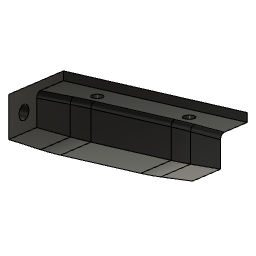
Back mount attachment (Autodesk Fusion 360 archive; units mm, degrees)
design "Back mount attachment" references "Micro Delta Rework", "Plaque de support"
Autodesk Fusion 360 part; units mm, degrees
note: some values were not read from the file. Set by a fixed rule: which face or edge a step refers to.
derive "Dérivé à partir de Micro Delta Rework v14" from "Micro Delta Rework v14"
derive "Dérivé à partir de Plaque de support v19" from "Plaque de support v19"
box "BoitePrimitive1" add length 25 width 25 height 110 placed x (0, 1, 0) y (-1, 0, 0) z (0, 0, 1) at (25, 0, 0)
hole "Perçage1" at (12.5, 12.5, 110) direction (0, 0, -1) diameter 8.2 end through all
sketch "Esquisse8" plane through (25, 0, 0) normal (1, 0, 0) x (0, 0, -1)
  line L0 (-110, 0) -> (0, 0)
  line L1 (0, 0) -> (0, 25)
  line L2 (0, 25) -> (-110, 25)
  line L3 (-110, 25) -> (-110, 0)
  line L4 (-110, 20) -> (0, 20)
  dimension "base_l" = 25
  dimension "tige_diam" = 8
  dimension "tige_jeu" = 0.2
  dimension "fixation_ep" = 5
  dimension "fixation_prof" = 20
  dimension "vis_diam" = 6
  dimension "vis_jeu" = 0.6
  dimension "plaque0_l1_Ref" = 160
  dimension "plaque0_l2_Ref" = 95
  dimension "plaque0_l1_Ref_Ref" = 160
  dimension "plaque0_l2_Ref_Ref" = 95
  dimension "support_chanf_Ref" = 25
  dimension "d43" = 5
  dimension "haut_ep_Ref" = 17
  dimension "plaque_ep_Ref" = 2.1
  dimension "haut_conge_Ref" = 3
  constraint coincident L3 L4.start
  constraint coincident L1 L4.end
  constraint perpendicular L1 L4
  measures "d43" distance of L2 L4
extrude "Extrusion2" add sketch "Esquisse8" along normal blind 20 contours L1 L2 L3 L4
sketch "Esquisse9" plane through (0, 20, 0) normal (0, -1, 0) x (1, 0, 0)
  line L0 (25, 110) -> (25, 0)
  line L1 (25, 0) -> (45, 0)
  line L2 (45, 0) -> (45, 110)
  line L3 (45, 110) -> (25, 110)
  line L4 (45, 55) -> (25, 55) construction
  line L5 (25, 110) -> (45, 55) construction
  line L6 (45, 110) -> (25, 55) construction
  line L7 (25, 55) -> (45, 0) construction
  line L8 (45, 55) -> (25, 0) construction
  circle A0 centre (35, 82.5) radius 3.3
  circle A1 centre (35, 27.5) radius 3.3
  dimension "d46" = 6.6
  dimension "d47" = 6.6
  constraint midpoint L2 L4.start
  constraint midpoint L0 L4.end
  constraint coincident L0.start L3.end
  constraint coincident L2.end L3.start
  constraint coincident L1.end L2.start
  constraint coincident L0.end L1.start
  constraint midpoint L5 A0.centre
  constraint midpoint L8 A1.centre
  measures "d46" diameter of A0
  measures "d47" diameter of A1
extrude "Extrusion3" cut sketch "Esquisse9" against normal through all contours A0 | A1
chamfer "Chanfrein5" distance 2 distance2 25 4 edges at (25, 10, 110) (25, 10, 0) (12.5, 0, 110) (12.5, 0, 0) measured on face at (2.8038, 12.6021, 110) measured on face at (2.8038, 12.3979, 0) measured on face at (2.8038, 12.6021, 110) measured on face at (2.8038, 12.3979, 0)
fillet "Congé3" radius 150 4 edges at (25, 10, 85) (12.5, 0, 85) (25, 10, 25) (12.5, 0, 25)
fillet "Congé4" radius 3 5 edges at (23.7611, 20, 9.5143) (24.8805, 20, 25.0048) (25, 20, 55) (24.8805, 20, 84.9952) (23.7611, 20, 100.4857)
equation "base_l = 25 mm"
equation "d4 = plaque0_l1_Ref - support_chanf_Ref * 2"
equation "tige_diam = 8 mm"
equation "tige_jeu = 0.2 mm"
equation "d10 = tige_diam + tige_jeu"
equation "fixation_ep = 5 mm"
equation "fixation_prof = 20 mm"
equation "vis_diam = 6 mm"
equation "vis_jeu = 0.6 mm"
equation "d43 = fixation_ep"
equation "d44 = fixation_prof"
equation "d46 = vis_diam + vis_jeu"
equation "d47 = vis_diam + vis_jeu"
equation "d50 = base_l"
named bodies: "Back mount attachment"

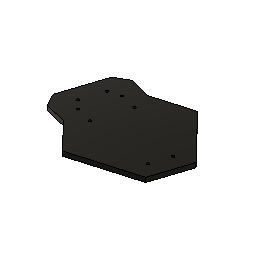
design "Plaque de support" references "Micro Delta Rework"
Autodesk Fusion 360 part; units mm, degrees
derive "Dérivé à partir de Micro Delta Rework v14" from "Micro Delta Rework v14"
sketch "Esquisse1" plane through (0, 0, 0) normal (0, 1, 0) x (1, 0, 0)
  line L0 (0, 0) -> (160, 0)
  line L1 (0, 0) -> (-47.5, 82.2724)
  line L2 (0, 0) -> (95, 0) construction
  line L3 (-47.5, 82.2724) -> (32.5, 220.8365)
  line L4 (-47.5, 82.2724) -> (112.5, 82.2724) construction
  line L5 (160, 0) -> (207.5, 82.2724)
  line L6 (160, 0) -> (255, 0) construction
  line L7 (207.5, 82.2724) -> (127.4604, 220.8136)
  line L8 (207.5, 82.2724) -> (367.5, 82.2724) construction
  line L9 (127.4604, 220.8136) -> (32.5, 220.8365)
  dimension "d3" = 160
  dimension "d4" = 120
  dimension "d5" = 95
  dimension "d6" = 60
  dimension "d7" = 160
  dimension "d8" = 60
  dimension "d9" = 95
  dimension "d10" = 120.016
  dimension "d11" = 160
  constraint coincident L0.start L1.start
  constraint horizontal L0
  constraint horizontal L2
  constraint horizontal L4
  constraint horizontal L6
  constraint horizontal L8
  measures "d3" distance of L0.start L0.end
  measures "d4" angle of L1 L2
  measures "d5" distance of L0.start L1.end
  measures "d6" angle of L3 L4
  measures "d7" distance of L1.end L3.end
  measures "d8" angle of L5 L6
  measures "d9" distance of L0.end L5.end
  measures "d10" angle of L7 L8
  measures "d11" distance of L5.end L7.end
extrude "Extrusion1" add sketch "Esquisse1" along normal blind 10.12
extrude "Extrusion2" add 1 faces at (-20.8333, 3.3733, -128.4604) along direction (-0.866025, 0, -0.5) blind 80
chamfer "Chanfrein1" distance 25 angle 45 2 edges at (-36.782, 5.06, -260.8365) (-116.782, 5.06, -122.2724)
sketch "Esquisse2" plane through (0, 10.12, 0) normal (0, 1, 0) x (-1, 0, 0)
  line L0 (104.282, -143.923) -> (95.1314, -109.7724)
  line L1 (95.1314, -109.7724) -> (47.5, -82.2724)
  line L2 (47.5, -82.2724) -> (0, 0)
  line L3 (0, 0) -> (-160, 0)
  line L4 (-160, 0) -> (-207.5, -82.2724)
  line L5 (-207.5, -82.2724) -> (-127.4604, -220.8136)
  line L6 (-127.4604, -220.8136) -> (-32.5, -220.8365)
  line L7 (-32.5, -220.8365) -> (15.1314, -248.3365)
  line L8 (15.1314, -248.3365) -> (49.282, -239.1858)
  line L9 (49.282, -239.1858) -> (104.282, -143.923)
  line L10 (97.782, -155.1814) -> (-162.75, -4.7631) construction
  line L11 (55.782, -227.9275) -> (-204.75, -77.5093) construction
  line L12 (-15.1795, -230.8365) -> (64.8205, -92.2724) construction
  circle A0 centre (45.8205, -125.1814) radius 3.025
  circle A1 centre (3.8205, -197.9275) radius 3.025
  line L13 (-63.4246, -231.3994) -> (35.087, -60.7724) construction
  circle A2 centre (9.8805, -104.4314) radius 3.025
  circle A3 centre (-32.1195, -177.1775) radius 3.025
  line L14 (6.4495, -243.324) -> (86.4495, -104.7599) construction
  line L15 (90.5195, -167.7604) -> (-170.0125, -17.3422) construction
  line L16 (63.0445, -215.3485) -> (-197.4875, -64.9303) construction
  circle A4 centre (60.187, -150.2479) radius 3.025
  circle A5 centre (32.712, -197.836) radius 3.025
  line L17 (76.782, -191.5544) -> (-183.75, -41.1362) construction
  line L18 (-119.5855, 0) -> (-187.2861, -117.2609) construction
  line L19 (-160, 0) -> (-153.4358, -58.6304) construction
  line L20 (-153.4358, -58.6304) -> (-207.5, -82.2724) construction
  line L21 (-160, 0) -> (-129.6891, -17.5) construction
  line L22 (-207.5, -82.2724) -> (-177.1891, -99.7724) construction
  line L23 (-177.1891, -99.7724) -> (-183.75, -41.1362) construction
  line L24 (-183.75, -41.1362) -> (-129.6891, -17.5) construction
  line L25 (-156.7196, -29.3181) -> (-141.5641, -38.0681) construction
  line L26 (-180.4679, -70.4514) -> (-165.3124, -79.2014) construction
  circle A6 centre (-141.5641, -38.0681) radius 3.025
  circle A7 centre (-165.3124, -79.2014) radius 3.025
  dimension "d24" = 38
  dimension "d26" = 38
  dimension "d28" = 60
  dimension "d30" = 6.05
  dimension "d31" = 6.05
  dimension "d39" = 41.5
  dimension "d40" = 6.05
  dimension "d43" = 6.05
  dimension "d46" = 35.025
  dimension "d49" = 27.525
  dimension "d50" = 27.525
  dimension "d51" = 6.05
  dimension "d52" = 6.05
  dimension "d53" = 35
  dimension "d54" = 6.05
  dimension "d55" = 6.05
  constraint coincident L9 L10.start
  constraint coincident L4 L10.end
  constraint perpendicular L4 L10
  constraint coincident L9 L11.start
  constraint coincident L4 L11.end
  constraint perpendicular L4 L11
  constraint coincident L7 L12.start
  constraint coincident L1 L12.end
  constraint perpendicular L1 L12
  constraint coincident L10 A0.centre
  constraint coincident L12 A0.centre
  constraint coincident L12 A1.centre
  constraint coincident L11 A1.centre
  constraint coincident L2 L13.end
  constraint parallel L12 L13
  constraint coincident L13 A2.centre
  constraint coincident L10 A2.centre
  constraint coincident L11 A3.centre
  constraint coincident L13 A3.centre
  constraint coincident L7 L14.start
  constraint coincident L1 L14.end
  constraint perpendicular L1 L14
  constraint coincident L9 L15.start
  constraint coincident L4 L15.end
  constraint perpendicular L4 L15
  constraint coincident L9 L16.start
  constraint coincident L4 L16.end
  constraint perpendicular L4 L16
  constraint coincident L14 A4.centre
  constraint coincident L15 A4.centre
  constraint coincident L14 A5.centre
  constraint coincident L16 A5.centre
  constraint midpoint L9 L17.start
  constraint midpoint L4 L17.end
  constraint coincident L3 L18.start
  constraint coincident L5 L18.end
  constraint parallel L4 L18
  constraint coincident L3.end L4.start
  constraint midpoint L18 L19.end
  constraint coincident L4.end L5.start
  constraint coincident L18 L21.end
  constraint perpendicular L18 L21
  constraint coincident L18 L22.end
  constraint perpendicular L18 L22
  constraint midpoint L24 L25.start
  constraint coincident L18 L25.end
  constraint perpendicular L18 L25
  constraint midpoint L20 L26.start
  constraint coincident L18 L26.end
  constraint perpendicular L18 L26
  constraint coincident L25.end A6.centre
  constraint coincident L26.end A7.centre
  measures "d24" distance of L1 L10
  measures "d26" distance of L7 L11
  measures "d28" distance of L9 L12
  measures "d30" diameter of A0
  measures "d31" diameter of A1
  measures "d39" distance of L12 L13
  measures "d40" diameter of A2
  measures "d43" diameter of A3
  measures "d46" distance of L9 L14
  measures "d49" distance of L0.start L15
  measures "d50" distance of L8.end L16
  measures "d51" diameter of A4
  measures "d52" diameter of A5
  measures "d53" distance of L4 L18
  measures "d54" diameter of A6
  measures "d55" diameter of A7
extrude "Extrusion3" cut sketch "Esquisse2" against normal through all contours A0 | A1 | A2 | A3 | A4 | A5 | A6 | A7
equation "plaque0_l1_Ref = 160 mm"
equation "plaque0_l2_Ref = 95 mm"
equation "d3 = plaque0_l1_Ref"
equation "d5 = plaque0_l2_Ref"
equation "d7 = plaque0_l1_Ref"
equation "d9 = plaque0_l2_Ref"
equation "d11 = plaque0_l1_Ref"
equation "plaque_ep = 10.12 mm"
equation "d13 = plaque_ep"
equation "d15 = support_prof"
equation "d17 = support_chanf"
equation "support_prof = 80 mm"
equation "support_chanf = 25 mm"
equation "haut_ep_Ref = 17 mm"
equation "plaque_ep_Ref = 2.1 mm"
equation "haut_conge_Ref = 3 mm"
equation "d24 = trou_butée_x"
equation "trou_butée_x = 38 mm"
equation "d26 = trou_butée_x"
equation "trou_butée_y = 60 mm"
equation "d28 = trou_butée_y"
equation "trou_diam = 6.05 mm"
equation "d30 = trou_diam"
equation "d31 = trou_diam"
equation "trou_butée_entraxe = 41.5 mm"
equation "d39 = trou_butée_entraxe"
equation "d40 = trou_diam"
equation "d43 = trou_diam"
equation "trou_glissière_y = 35.025 mm"
equation "trou_glissière_entraxe = 55 mm"
equation "d46 = trou_glissière_y"
equation "trou_glissière_x = 27.525 mm"
equation "d49 = trou_glissière_x"
equation "d50 = trou_glissière_x"
equation "d51 = trou_diam"
equation "d52 = trou_diam"
equation "d54 = trou_diam"
equation "d55 = trou_diam"

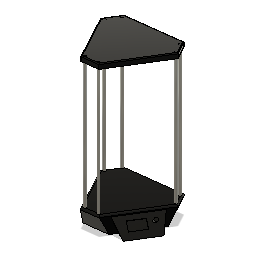
design "Micro Delta Rework"
Autodesk Fusion 360 part; units mm, degrees
sketch "Esquisse1" plane through (0, 0, 0) normal (0, 1, 0) x (1, 0, 0)
  line L0 (0, 0) -> (160, 0)
  line L1 (0, 0) -> (-47.5, 82.2724)
  line L2 (0, 0) -> (95, 0) construction
  line L3 (160, 0) -> (207.5, 82.2724)
  line L4 (160, 0) -> (255, 0) construction
  line L5 (-47.5, 82.2724) -> (32.5, 220.8365)
  line L6 (-47.5, 82.2724) -> (112.5, 82.2724) construction
  line L7 (207.5, 82.2724) -> (127.5, 220.8365)
  line L8 (207.5, 82.2724) -> (367.5, 82.2724) construction
  line L9 (127.5, 220.8365) -> (32.5, 220.8365)
  line L10 (-7.5, 151.5544) -> (183.75, 41.1362) construction
  line L11 (80, 0) -> (80, 220.8365) construction
  line L12 (25, -46) -> (135, -46) construction
  line L13 (5, 0) -> (155, 0)
  circle A0 centre (3.4641, 26) radius 6
  circle A1 centre (156.5359, 26) radius 6
  circle A2 centre (183.2513, 72.2724) radius 6
  circle A3 centre (106.7154, 204.8365) radius 6
  circle A4 centre (53.2846, 204.8365) radius 6
  circle A5 centre (-23.2513, 72.2724) radius 6
  line L14 (18.4752, 0) -> (-38.2624, 98.2724) construction
  line L15 (135.9202, -9.7075) -> (198.2624, 98.2724) construction
  line L16 (23.2624, 204.8365) -> (136.7376, 204.8365) construction
  line L17 (-15.0111, 26) -> (175.0111, 26) construction
  line L18 (192.4889, 56.2724) -> (97.4778, 220.8365) construction
  line L19 (-32.4889, 56.2724) -> (62.5222, 220.8365) construction
  point P0 (80, 101.0363)
  point P1 (80, 0)
  point P2 (80, -46)
  dimension "d1" = 160
  dimension "d2" = 120
  dimension "d3" = 95
  dimension "d4" = 95
  dimension "d5" = 60
  dimension "d6" = 60
  dimension "d7" = 160
  dimension "d8" = 120
  dimension "d9" = 160
  dimension "d62" = 110
  dimension "d63" = 150
  dimension "d64" = 46
  dimension "d98" = 12
  dimension "d99" = 12
  dimension "d100" = 12
  dimension "d101" = 12
  dimension "d102" = 12
  dimension "d103" = 12
  dimension "d104" = 16
  dimension "d105" = 16
  dimension "d106" = 16
  dimension "d107" = 26
  dimension "d108" = 26
  dimension "d109" = 26
  constraint coincident L0.start L1.start
  constraint horizontal L0
  constraint horizontal L2
  constraint horizontal L4
  constraint horizontal L6
  constraint horizontal L8
  constraint midpoint L5 L10.start
  constraint midpoint L3 L10.end
  constraint midpoint L0 P1
  constraint midpoint L9 L11.end
  constraint coincident L11 P0
  constraint coincident L10 P0
  constraint horizontal L12
  constraint horizontal L13
  constraint midpoint L13 P1
  constraint coincident L11 P1
  constraint midpoint L12 P2
  constraint coincident L11 P2
  constraint collinear L0 L13
  constraint coincident L2 L14.start
  constraint coincident L5 L14.end
  constraint coincident L7 L15.end
  constraint coincident L5 L16.start
  constraint coincident L7 L16.end
  constraint parallel L9 L16
  constraint parallel L1 L14
  constraint parallel L3 L15
  constraint coincident L1 L17.start
  constraint coincident L3 L17.end
  constraint coincident L3 L18.start
  constraint coincident L9 L18.end
  constraint coincident L1 L19.start
  constraint coincident L9 L19.end
  constraint parallel L0 L17
  constraint parallel L7 L18
  constraint parallel L5 L19
  constraint coincident A0.centre L17
  constraint coincident A0.centre L14
  constraint coincident A5.centre L14
  constraint coincident A5.centre L19
  constraint coincident A4.centre L19
  constraint coincident A4.centre L16
  constraint coincident A3.centre L18
  constraint coincident A3.centre L16
  constraint coincident A1.centre L15
  constraint coincident A1.centre L17
  constraint coincident A2.centre L18
  constraint coincident A2.centre L15
  measures "d1" distance of L0.start L0.end
  measures "d2" angle of L1 L2
  measures "d3" distance of L0.start L1.end
  measures "d4" distance of L0.end L3.end
  measures "d5" angle of L3 L4
  measures "d6" angle of L5 L6
  measures "d7" distance of L1.end L5.end
  measures "d8" angle of L7 L8
  measures "d9" distance of L3.end L7.end
  measures "d62" distance of L12.start L12.end
  measures "d63" distance of L13.start L13.end
  measures "d64" distance of L12 L13
  measures "d98" diameter of A0
  measures "d99" diameter of A1
  measures "d100" diameter of A2
  measures "d101" diameter of A3
  measures "d102" diameter of A4
  measures "d103" diameter of A5
  measures "d104" distance of L1 L14
  measures "d105" distance of L3 L15
  measures "d106" distance of L9 L16
  measures "d107" distance of L2 L17
  measures "d108" distance of L7 L18
  measures "d109" distance of L5 L19
ref_plane "Plan de construction1" through (0, 60, 0) normal (0, 1, 0) x (0, 0, 1)
sketch "Esquisse2" plane through (0, 60, 0) normal (0, 1, 0) x (1, 0, 0)
  line L0 (-30, 0) -> (190, 0)
  line L1 (-30, 0) -> (-62.5, 56.2917)
  line L2 (-30, 0) -> (35, 0) construction
  line L3 (-62.5, 56.2917) -> (47.5, 246.8172)
  line L4 (-62.5, 56.2917) -> (157.5, 56.2917) construction
  line L5 (190, 0) -> (222.5, 56.2917)
  line L6 (190, 0) -> (255, 0) construction
  line L7 (222.5, 56.2917) -> (112.5, 246.8172)
  line L8 (222.5, 56.2917) -> (442.5, 56.2917) construction
  line L9 (112.5, 246.8172) -> (47.5, 246.8172)
  line L10 (206.25, 28.1458) -> (-7.5, 151.5544) construction
  line L11 (80, 0) -> (80, 246.8172) construction
  line L12 (-56.7265, 66.2917) -> (-18.453, 0) construction
  line L13 (41.7265, 236.8172) -> (118.2735, 236.8172) construction
  line L14 (178.453, 0) -> (216.7265, 66.2917) construction
  circle A0 centre (-25.3812, 12) radius 5
  circle A1 centre (-49.7983, 54.2917) radius 5
  circle A2 centre (184.0544, 9.702) radius 5
  circle A3 centre (206.8348, 49.1587) radius 5
  circle A4 centre (55.5829, 236.8172) radius 5
  circle A5 centre (104.4171, 236.8172) radius 5
  point P0 (80, 101.0363)
  point P1 (80, 101.0363)
  dimension "d18" = 220
  dimension "d19" = 120
  dimension "d20" = 65
  dimension "d21" = 60
  dimension "d22" = 220
  dimension "d23" = 60
  dimension "d24" = 65
  dimension "d25" = 120
  dimension "d26" = 220
  dimension "d43" = 10
  dimension "d44" = 10
  dimension "d45" = 10
  dimension "d47" = 10
  dimension "d48" = 10
  dimension "d49" = 10
  dimension "d50" = 10
  dimension "d51" = 10
  dimension "d52" = 10
  dimension "d53" = 12
  dimension "d54" = 12
  dimension "d55" = 12
  dimension "d56" = 12
  constraint horizontal L0
  constraint horizontal L2
  constraint horizontal L4
  constraint horizontal L6
  constraint horizontal L8
  constraint midpoint L5 L10.start
  constraint midpoint L3 L10.end
  constraint midpoint L0 L11.start
  constraint midpoint L9 L11.end
  constraint coincident L10 P1
  constraint coincident L11 P1
  constraint coincident P1 P0
  constraint coincident L3 L12.start
  constraint coincident L2 L12.end
  constraint coincident L3 L13.start
  constraint coincident L7 L13.end
  constraint coincident L0 L14.start
  constraint coincident L7 L14.end
  constraint parallel L1 L12
  constraint parallel L9 L13
  constraint parallel L5 L14
  constraint coincident L12 A0.centre
  constraint coincident L12 A1.centre
  constraint coincident L14 A2.centre
  constraint coincident L14 A3.centre
  constraint coincident L13 A4.centre
  constraint coincident L13 A5.centre
  measures "d18" distance of L0.start L0.end
  measures "d19" angle of L1 L2
  measures "d20" distance of L0.start L1.end
  measures "d21" angle of L3 L4
  measures "d22" distance of L1.end L3.end
  measures "d23" angle of L5 L6
  measures "d24" distance of L0.end L5.end
  measures "d25" angle of L7 L8
  measures "d26" distance of L5.end L7.end
  measures "d43" distance of L1 L12
  measures "d44" distance of L5 L14
  measures "d45" distance of L9 L13
  measures "d47" diameter of A0
  measures "d48" diameter of A1
  measures "d49" diameter of A2
  measures "d50" diameter of A3
  measures "d51" diameter of A4
  measures "d52" diameter of A5
  measures "d53" distance of L3 A4.centre
  measures "d54" distance of L7 A5.centre
  measures "d55" distance of L2 A0.centre
  measures "d56" distance of L3 A1.centre
loft "Lissage1" add profiles "Esquisse1", "Esquisse2" section 1 contours L0 L1 L3 L5 L7 L9 L13 | A0 | A1 | A2 | A3 | A4 | A5 section 2 contours L0 L1 L3 L5 L7 L9 | A0 | A1 | A2 | A3 | A4 | A5 makes body 1
ref_plane "Plan de construction2" through (80, 490, -123.4086) normal (0, 1, 0) x (0, 0, 1)
sketch "Esquisse3" plane through (80, 490, -123.4086) normal (0, 1, 0) x (1, 0, 0)
  line L0 (-107.5, -121.9652) -> (107.5, -121.9652)
  line L1 (-107.5, -121.9652) -> (-140, -65.6736)
  line L2 (-107.5, -121.9652) -> (-42.5, -121.9652) construction
  line L3 (-140, -65.6736) -> (-32.5, 120.5219)
  line L4 (-140, -65.6736) -> (75, -65.6736) construction
  line L5 (107.5, -121.9652) -> (140, -65.6736)
  line L6 (107.5, -121.9652) -> (172.5, -121.9652) construction
  line L7 (140, -65.6736) -> (32.5, 120.5219)
  line L8 (140, -65.6736) -> (355, -65.6736) construction
  line L9 (32.5, 120.5219) -> (-32.5, 120.5219)
  line L10 (123.75, -93.8194) -> (-86.25, 27.4241) construction
  line L11 (0, -121.9652) -> (0, 120.5219) construction
  point P0 (0, -22.3723)
  point P1 (0, -22.3723)
  dimension "d28" = 215
  dimension "d29" = 120
  dimension "d30" = 65
  dimension "d31" = 60
  dimension "d32" = 215
  dimension "d33" = 60
  dimension "d34" = 65
  dimension "d35" = 120
  dimension "d36" = 215
  constraint horizontal L0
  constraint horizontal L2
  constraint horizontal L4
  constraint horizontal L6
  constraint horizontal L8
  constraint midpoint L5 L10.start
  constraint midpoint L3 L10.end
  constraint midpoint L0 L11.start
  constraint midpoint L9 L11.end
  constraint coincident L11 P1
  constraint coincident L10 P1
  constraint coincident P1 P0
  measures "d28" distance of L0.start L0.end
  measures "d29" angle of L1 L2
  measures "d30" distance of L0.start L1.end
  measures "d31" angle of L3 L4
  measures "d32" distance of L1.end L3.end
  measures "d33" angle of L5 L6
  measures "d34" distance of L0.end L5.end
  measures "d35" angle of L7 L8
  measures "d36" distance of L5.end L7.end
extrude "Extrusion1" add sketch "Esquisse3" along normal blind 17 separate body makes body 2
fillet "Congé1" radius 3 6 edges at (166.25, 507, -150.8328) (80, 507, -243.9305) (-6.25, 507, -150.8328) (-43.75, 507, -29.5892) (80, 507, -1.4434) (203.75, 507, -29.5892) on bodies 2
shell "Coque1" thickness 2.1 removed faces 1 at (69.1667, 490, -119.8002) on bodies 2
extrude "Extrusion2" add sketch "Esquisse2" along normal up to surface (444.9 mm away) separate body contours A0 | A1 | A2 | A3 | A4 | A5 makes body 3 at (52.5971, 356.6, -240.8279) makes body 4 at (182.074, 356.6, -5.1109) makes body 5 at (-44.8321, 208.3, -53.7112) makes body 6 at (109.3833, 208.3, -236.2368) makes body 7 at (211.801, 208.3, -48.5782) makes body 8 at (-20.415, 208.3, -11.4195)
sketch "Esquisse8" plane through (0, 0, 0) normal (0, 0, 1) x (1, 0, 0)
  line L0 (0, 0) -> (160, 0)
  line L1 (160, 0) -> (190, 60)
  line L2 (190, 60) -> (-30, 60)
  line L3 (-30, 60) -> (0, 0)
  line L4 (-30, 60) -> (190, 60) construction
  line L5 (5, 51) -> (155, 51)
  line L6 (80, 60) -> (80, 0) construction
  line L7 (25, 0) -> (135, 0)
  line L8 (25, 0) -> (5, 51)
  line L9 (135, 0) -> (155, 51)
  point P0 (80, 51)
  dimension "d69" = 150
  dimension "d70" = 9
  constraint horizontal L5
  constraint midpoint L2 L6.start
  constraint midpoint L0 L6.end
  constraint midpoint L5 P0
  constraint coincident L6 P0
  constraint coincident L7.start L8.start
  constraint coincident L7.end L9.start
  measures "d69" distance of L5.start L5.end
  measures "d70" distance of L4 L5
ref_plane "Plan de construction4" through (5, 51, 0) normal (0, 0.669769, 0.74257) x (-1, 0, 0)
sketch "Esquisse10" plane through (5, 51, 0) normal (0, 0.669769, 0.74257) x (-1, 0, 0)
  line L0 (0, 0) -> (-150, 0)
  line L1 (-20, 68.6804) -> (-130, 68.6804)
  line L2 (0, 0) -> (-20, 68.6804)
  line L3 (-130, 68.6804) -> (-150, 0)
  line L4 (-38, 16) -> (-93, 16)
  line L5 (-93, 16) -> (-93, 46)
  line L6 (-93, 46) -> (-38, 46)
  line L7 (-38, 46) -> (-38, 16)
  circle A0 centre (-114, 26) radius 6
  dimension "d76" = 55
  dimension "d77" = 30
  dimension "d78" = 12
  dimension "d87" = 16
  dimension "d88" = 38
  dimension "d89" = 26
  dimension "d90" = 36
  constraint coincident L0.start L2.start
  constraint coincident L1.start L2.end
  constraint coincident L1.end L3.start
  constraint coincident L0.end L3.end
  constraint horizontal L4
  constraint vertical L5
  constraint horizontal L6
  constraint vertical L7
  measures "d76" distance of L4.start L4.end
  measures "d77" distance of L4.start L6.end
  measures "d78" diameter of A0
  measures "d87" distance of L0 L4
  measures "d88" distance of L0.start L7
  measures "d89" distance of L0 A0.centre
  measures "d90" horizontal distance of L0.end A0.centre
loft "Lissage2" add profiles "Esquisse8", "Esquisse10" section 1 contours L0 L5 L7 L8 L9 section 2 contours L0 L1 L2 L3 | L4 L5 L6 L7 | A0 separate body makes body 9
fillet "Congé2" radius 6 6 edges at (167.5, 60, -151.5544) (206.25, 60, -28.1458) (80, 60, 0) (-46.25, 60, -28.1458) (-7.5, 60, -151.5544) (80, 60, -246.8172) on bodies 1
extrude "Extrusion3" cut sketch "Esquisse10" against normal blind 3 contours L4 L5 L6 L7 bodies 9
extrude "Extrusion4" add sketch "Esquisse10" along normal blind 15 contours A0 bodies 9
extrude "Extrusion5" add sketch "Esquisse1" against normal blind 3.6 contours A0 | A1 | A2 | A3 | A4 | A5 bodies 1
equation "d1 = plaque0_l1"
equation "d3 = plaque0_l2"
equation "d4 = plaque0_l2"
equation "d7 = plaque0_l1"
equation "d9 = plaque0_l1"
equation "plaque0_l1 = 160 mm"
equation "plaque0_l2 = 95 mm"
equation "plaque1_l1 = 220 mm"
equation "plaque1_l2 = 65 mm"
equation "plaque3_l1 = 215 mm"
equation "plaque3_l2 = 65 mm"
equation "base_haut = 60 mm"
equation "d17 = base_haut"
equation "d18 = plaque1_l1"
equation "d20 = plaque1_l2"
equation "d22 = plaque1_l1"
equation "d24 = plaque1_l2"
equation "d26 = plaque1_l1"
equation "d27 = tige_l"
equation "d28 = plaque3_l1"
equation "d30 = plaque3_l2"
equation "d32 = plaque3_l1"
equation "d34 = plaque3_l2"
equation "d36 = plaque3_l1"
equation "haut_ep = 17 mm"
equation "d38 = haut_ep"
equation "tige_dec_l1 = 12 mm"
equation "tige_dec_l2 = 10 mm"
equation "tige_l = 430 mm"
equation "d43 = tige_dec_l2"
equation "d44 = tige_dec_l2"
equation "d45 = tige_dec_l2"
equation "tige_diam = 10 mm"
equation "d47 = tige_diam"
equation "d48 = tige_diam"
equation "d49 = tige_diam"
equation "d50 = tige_diam"
equation "d51 = tige_diam"
equation "d52 = tige_diam"
equation "d53 = tige_dec_l1"
equation "d54 = tige_dec_l1"
equation "d55 = tige_dec_l1"
equation "d56 = tige_dec_l1"
equation "tableau_l1 = 150 mm"
equation "tableau_l2 = 110 mm"
equation "tableau_larg = 60 mm"
equation "d62 = tableau_l2"
equation "d63 = tableau_l1"
equation "d64 = tableau_base_dec_bas"
equation "tableau_base_dec_haut = 9 mm"
equation "tableau_base_dec_bas = 46 mm"
equation "d69 = tableau_l1"
equation "d70 = tableau_base_dec_haut"
equation "d72 = haut_conge"
equation "d75 = bas_conge"
equation "d76 = tableau_ecran_long"
equation "d77 = tableau_ecran_larg"
equation "d78 = tableau_bounton_diam"
equation "tableau_ecran_long = 55 mm"
equation "tableau_ecran_larg = 30 mm"
equation "tableau_ecran_x = 38 mm"
equation "tableau_ecran_y = 16 mm"
equation "tableau_bounton_diam = 12 mm"
equation "tableau_bounton_l = 15 mm"
equation "tableau_bounton_x = 36 mm"
equation "tableau_bounton_y = 26 mm"
equation "d87 = tableau_ecran_y"
equation "d88 = tableau_ecran_x"
equation "d89 = tableau_bounton_y"
equation "d90 = tableau_bounton_x"
equation "d93 = tableau_bounton_l"
equation "patin_dec_l1 = 26 mm"
equation "patin_dec_l2 = 16 mm"
equation "patin_diam = 12 mm"
equation "d98 = patin_diam"
equation "d99 = patin_diam"
equation "d100 = patin_diam"
equation "d101 = patin_diam"
equation "d102 = patin_diam"
equation "d103 = patin_diam"
equation "d104 = patin_dec_l2"
equation "d105 = patin_dec_l2"
equation "d106 = patin_dec_l2"
equation "d107 = patin_dec_l1"
equation "d108 = patin_dec_l1"
equation "d109 = patin_dec_l1"
equation "patin_ep = 3.6 mm"
equation "d111 = -patin_ep"
equation "plaque_ep = 2.1 mm"
equation "d114 = plaque_ep"
equation "haut_conge = 3 mm"
equation "bas_conge = 6 mm"
named bodies: "base", "haut", "tige5", "tige3", "tige2", "tige6", "tige4", "tige1", "tableau"
